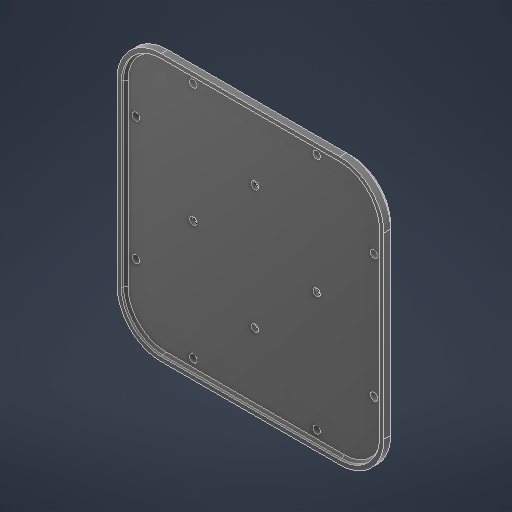
# Autodesk Inventor part: battery_pack_cover_rear
Saved by Autodesk Inventor 2026.1 (Build 301233000, 233)
## iProperties
Created: 2026-05-18
Part Number: battery_pack_cover_rear
Material: ABS Plastic
Document SubType Name: Modeling
Designer: aaron
Density: 1.06 g/cm^3
Appearance: Smooth - White
Author: aaron
Autodesk Inventor part; units mm, degrees
ref_plane "YZ Plane" through (0, 0, 0) normal (1, 0, 0) x (0, 1, 0)
ref_plane "XZ Plane" through (0, 0, 0) normal (0, 1, 0) x (-1, 0, 0)
ref_plane "XY Plane" through (0, 0, 0) normal (0, 0, 1) x (1, 0, 0)
sketch "Sketch1" plane through (0, 0, 0) normal (0, 0, 1) x (1, 0, 0)
  line L0 (20, 0) -> (101, 0)
  line L1 (121, 20) -> (121, 101)
  line L2 (101, 121) -> (20, 121)
  line L3 (0, 101) -> (0, 20)
  arc A0 (20, 121) -> (0, 101) centre (20, 101) ccw
  arc A1 (121, 101) -> (101, 121) centre (101, 101) ccw
  arc A2 (101, 0) -> (121, 20) centre (101, 20) ccw
  arc A3 (0, 20) -> (20, 0) centre (20, 20) ccw
  point P0 (0, 0)
  point P1 (121, 121)
  point P2 (121, 0)
  point P3 (0, 121)
  dimension "d0" = 121
  dimension "d1" = 121
  dimension "d2" = 20
  constraints: 8 end point, 8 point on circle, 8 point on line, 8 tangent, 4 centre point, 3 equal radius, 2 parallel, 1 horizontal, 1 perpendicular
  measures "d0" distance of point (121, 121) point (0, 121)
  measures "d1" distance of point (121, 0) point (121, 121)
  measures "d2" radius of A0
extrude "Extrusion1" add sketch "Sketch1" along normal blind 3
sketch "Sketch2" plane through (0, 0, 3) normal (0, 0, 1) x (1, 0, 0)
  arc A0 (101, 0) -> (121, 20) centre (101, 20) ccw projected
  line L0 (121, 20) -> (121, 101) projected
  arc A1 (121, 101) -> (101, 121) centre (101, 101) ccw projected
  line L1 (101, 121) -> (20, 121) projected
  arc A2 (20, 121) -> (0, 101) centre (20, 101) ccw projected
  line L2 (0, 101) -> (0, 20) projected
  arc A3 (0, 20) -> (20, 0) centre (20, 20) ccw projected
  line L3 (20, 0) -> (101, 0) projected
  line L4 (20, 119.05) -> (101, 119.05)
  arc A4 (119.05, 101) -> (101, 119.05) centre (101, 101) ccw
  line L5 (119.05, 101) -> (119.05, 20)
  arc A5 (101, 1.95) -> (119.05, 20) centre (101, 20) ccw
  line L6 (101, 1.95) -> (20, 1.95)
  arc A6 (1.95, 20) -> (20, 1.95) centre (20, 20) ccw
  line L7 (1.95, 20) -> (1.95, 101)
  arc A7 (20, 119.05) -> (1.95, 101) centre (20, 101) ccw
  point P0 (0, 0)
  dimension "d5" = 1.95
  constraints: 8 end point, 8 point on circle, 4 centre point, 7 other
  measures "d5" distance between parallel lines of L1 L4
extrude "Extrusion2" add sketch "Sketch2" along normal blind 2
chamfer "Chamfer1" distance 1 angle 45 8 edges at (1.95, 60.5, 3) (7.2367, 7.2367, 3) (60.5, 1.95, 3) (113.7633, 7.2367, 3) (119.05, 60.5, 3) (113.7633, 113.7633, 3) (60.5, 119.05, 3) (7.2367, 113.7633, 3)
sketch "Sketch3" plane through (0, 0, 0) normal (0, 0, -1) x (-1, 0, 0)
  circle A0 centre (-6.5, 88.5) radius 2.15 projected
  circle A1 centre (-6.5, 32.5) radius 2.15 projected
  circle A2 centre (-32.5, 6.5) radius 2.15 projected
  circle A3 centre (-88.5, 6.5) radius 2.15 projected
  circle A4 centre (-114.5, 32.5) radius 2.15 projected
  circle A5 centre (-114.5, 88.5) radius 2.15 projected
  circle A6 centre (-88.5, 114.5) radius 2.15 projected
  circle A7 centre (-32.5, 114.5) radius 2.15 projected
  circle A8 centre (-60.5, 60.5) radius 2.15 projected
  circle A9 centre (-60.5, 88.5) radius 2.15 projected
  circle A10 centre (-88.5, 60.5) radius 2.15 projected
  circle A11 centre (-60.5, 32.5) radius 2.15 projected
  circle A12 centre (-32.5, 60.5) radius 2.15 projected
  circle A13 centre (-88.5, 114.5) radius 1.65
  circle A14 centre (-32.5, 114.5) radius 1.65
  circle A15 centre (-60.5, 88.5) radius 1.65
  circle A16 centre (-114.5, 88.5) radius 1.65
  circle A17 centre (-88.5, 60.5) radius 1.65
  circle A18 centre (-60.5, 60.5) radius 1.65
  circle A19 centre (-32.5, 60.5) radius 1.65
  circle A20 centre (-6.5, 88.5) radius 1.65
  circle A21 centre (-6.5, 32.5) radius 1.65
  circle A22 centre (-60.5, 32.5) radius 1.65
  circle A23 centre (-114.5, 32.5) radius 1.65
  circle A24 centre (-88.5, 6.5) radius 1.65
  circle A25 centre (-32.5, 6.5) radius 1.65
  point P0 (0, 0)
  dimension "d11" = 3.3
  dimension "d12" = 3.3
  dimension "d13" = 3.3
  dimension "d14" = 3.3
  dimension "d15" = 3.3
  dimension "d16" = 3.3
  dimension "d17" = 3.3
  dimension "d18" = 3.3
  dimension "d19" = 3.3
  dimension "d20" = 3.3
  dimension "d21" = 3.3
  dimension "d22" = 3.3
  dimension "d23" = 3.3
  constraints: 13 centre point, 13 coincident
  measures "d11" diameter of A13
  measures "d12" diameter of A14
  measures "d13" diameter of A16
  measures "d14" diameter of A17
  measures "d15" diameter of A18
  measures "d16" diameter of A15
  measures "d17" diameter of A19
  measures "d18" diameter of A20
  measures "d19" diameter of A21
  measures "d20" diameter of A22
  measures "d21" diameter of A23
  measures "d22" diameter of A24
  measures "d23" diameter of A25
extrude "Extrusion3" cut sketch "Sketch3" against normal through all contours A13 | A14 | A15 | A16 | A17 | A19 | A20 | A21 | A22 | A23 | A24 | A25
chamfer "Chamfer2" distance 1.8 angle 45 4 edges at (62.15, 88.5, 0) (90.15, 60.5, 0) (34.15, 60.5, 0) (62.15, 32.5, 0)
chamfer "Chamfer3" distance 2 angle 45 8 edges at (60.5, 121, 0) (5.8579, 115.1421, 0) (0, 60.5, 0) (5.8579, 5.8579, 0) (60.5, 0, 0) (115.1421, 5.8579, 0) (121, 60.5, 0) (115.1421, 115.1421, 0)
sketch "Sketch4" plane through (0, 0, 0) normal (0, 0, -1) x (-1, 0, 0)
  line L0 (-53.168, 55.5218) -> (-59.1357, 52.7365)
  line L1 (-59.1357, 52.7365) -> (-65.1751, 55.2519)
  line L2 (-65.1751, 55.2519) -> (-59.2074, 58.0372)
  line L3 (-59.2074, 58.0372) -> (-53.168, 55.5218)
  line L4 (-53.168, 59.4718) -> (-59.2074, 61.9872)
  line L5 (-59.2074, 61.9872) -> (-59.2074, 64.5372)
  line L6 (-59.2074, 64.5372) -> (-65.1751, 61.7519)
  line L7 (-65.1751, 61.7519) -> (-65.1751, 58.5019)
  line L8 (-53.168, 59.4718) -> (-53.168, 58.7718)
  line L9 (-53.168, 58.7718) -> (-59.2074, 61.2872)
  line L10 (-59.2074, 61.2872) -> (-65.1751, 58.5019)
  line L11 (-59.2074, 69.1872) -> (-65.1751, 66.359)
  line L12 (-59.2074, 65.9372) -> (-59.2074, 68.4872)
  line L13 (-53.1419, 63.4218) -> (-59.2074, 65.9372)
  line L14 (-53.1419, 63.4218) -> (-53.1419, 62.7218)
  line L15 (-53.1419, 62.7218) -> (-59.1873, 65.2372)
  line L16 (-65.1751, 66.359) -> (-65.1751, 62.4519)
  line L17 (-59.1873, 65.2372) -> (-65.1751, 62.4519)
  line L18 (-59.2074, 69.1872) -> (-53.1419, 66.6718)
  line L19 (-53.1419, 66.6718) -> (-53.1419, 65.9718)
  line L20 (-53.1419, 65.9718) -> (-59.2074, 68.4872)
  point P0 (0, 0)
  dimension "d32" = 0.7
  dimension "d33" = 0.7
  dimension "d34" = 0.7
  dimension "d35" = 0.7
  dimension "d36" = 0
  dimension "d37" = 3.25
  dimension "d38" = 0.7
  dimension "d39" = 0.7
  dimension "d40" = 0.7
  dimension "d41" = 0.7
  dimension "d42" = 3.25
  dimension "d43" = 3.25
  dimension "d44" = 3.25
  dimension "d45" = 3.25
  dimension "d46" = 3.25
  dimension "d47" = 3.25
  constraints: 42 end point, 6 equal length, 5 parallel, 5 vertical, 2 collinear, 1 point on line
  measures "d32" distance of L13.start L15.start
  measures "d33" distance of L18.end L20.start
  measures "d34" distance of L4.start L9.start
  measures "d35" distance of L7.start L17.end
  measures "d36" horizontal distance of L3.start L9.end
  measures "d37" distance of L13.end L18.start
  measures "d38" distance of L9.end L4.end
  measures "d39" vertical distance of L5.end L15.end
  measures "d40" vertical distance of L15.end L13.end
  measures "d41" distance of L12.end L18.start
  measures "d42" vertical distance of L4.end L15.end
  measures "d43" distance of L13.start L18.end
  measures "d44" vertical distance of L4.start L15.start
  measures "d45" distance of L0.start L9.start
  measures "d46" distance of L1.end L7.end
  measures "d47" distance of L3.start L9.end
extrude "Extrusion4" cut sketch "Sketch4" against normal blind 0.001
equation "\"d1\" = d0"
equation "\"d12\" = d11"
equation "\"d13\" = d11"
equation "\"d14\" = d11"
equation "\"d15\" = d11"
equation "\"d16\" = d11"
equation "\"d17\" = d11"
equation "\"d18\" = d11"
equation "\"d19\" = d11"
equation "\"d20\" = d11"
equation "\"d21\" = d20"
equation "\"d22\" = d20"
equation "\"d23\" = d20"
equation "\"d33\" = d32"
equation "\"d34\" = d32"
equation "\"d38\" = d32"
equation "\"d39\" = d32"
equation "\"d40\" = d32"
equation "\"d41\" = d32"
equation "\"d42\" = d37"
equation "\"d44\" = d42"
equation "\"d45\" = d44"
equation "\"d46\" = d45"
equation "\"d47\" = d45"
body "Solid1"
